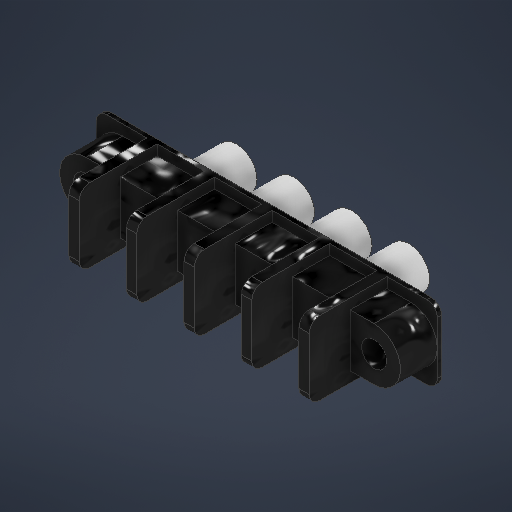
# Autodesk Inventor part: 52160004A
Saved by Autodesk Inventor 2026.2 (Build 302298010, 298A)
## iProperties
Created: 2026-08-03
Part Number: 52160004A
Material: Generic
Document SubType Name: Modeling
Designer: sonata
Density: 1 g/cm^3
Appearance: Default
Author: sonata
Autodesk Inventor part; units mm, degrees
ref_plane "YZ Plane" through (0, 0, 0) normal (1, 0, 0) x (0, 1, 0)
ref_plane "XZ Plane" through (0, 0, 0) normal (0, 1, 0) x (-1, 0, 0)
ref_plane "XY Plane" through (0, 0, 0) normal (0, 0, 1) x (1, 0, 0)
sketch "Sketch1" plane through (0, 0, 0) normal (0, 0, 1) x (1, 0, 0)
  line L0 (0, 0) -> (65.8, 0)
  line L1 (65.8, 0) -> (65.8, 14.2)
  line L2 (65.8, 14.2) -> (0, 14.2)
  line L3 (0, 14.2) -> (0, 0)
  dimension "d0" = 65.8
  dimension "d1" = 14.2
  constraints: 8 end point, 2 parallel, 1 coincident, 1 horizontal, 1 perpendicular
  measures "d0" distance of L1.end L2.end
  measures "d1" distance of L2.end L0.start
extrude "Extrusion1" add sketch "Sketch1" along normal blind 0.81
fillet "Fillet1" radius 2 4 edges at (0, 14.2, 0.405) (65.8, 14.2, 0.405) (65.8, 0, 0.405) (0, 0, 0.405)
sketch "Sketch2" plane through (0, 0, 0.81) normal (0, 0, 1) x (1, 0, 0)
  circle A0 centre (5.1, 7.1) radius 5.1
  line L0 (0, 12.2) -> (0, 2) projected
  circle A1 centre (60.7, 7.1) radius 5.1
  line L1 (65.8, 2) -> (65.8, 12.2) projected
  line L2 (5.1, 12.2) -> (60.7, 12.2)
  line L3 (60.7, 2) -> (5.1, 2)
  point P0 (0, 0)
  point P1 (0, 7.1)
  dimension "d5" = 10.2
  dimension "d6" = 10.2
  constraints: 5 tangent, 4 end point, 4 point on circle, 2 centre point, 2 horizontal alignment, 1 midpoint, 1 parallel
  measures "d5" diameter of A0
  measures "d6" diameter of A1
extrude "Extrusion2" add sketch "Sketch2" along normal blind 7.11
sketch "Sketch3" plane through (0, 0, 7.92) normal (0, 0, 1) x (1, 0, 0)
  line L0 (2, 0) -> (63.8, 0) projected
  line L1 (32.9, 0) -> (32.9, 14.2) construction
  line L2 (63.8, 14.2) -> (2, 14.2) projected
  circle A0 centre (5.1, 7.1) radius 2.4
  circle A1 centre (60.7, 7.1) radius 2.4
  line L3 (5.1, 7.1) -> (60.7, 7.1) construction
  point P0 (0, 0)
  dimension "d9" = 4.8
  dimension "d10" = 4.8
  dimension "d12" = 27.8
  dimension "d13" = 27.8
  dimension "d14" = 7.1
  constraints: 4 end point, 2 centre point, 2 midpoint, 1 horizontal
  measures "d9" diameter of A0
  measures "d10" diameter of A1
  measures "d12" distance from line of L1 L3.start
  measures "d13" distance from line of L3.end L1
  measures "d14" distance between parallel lines of L0 L3
extrude "Extrusion3" cut sketch "Sketch3" against normal through all
sketch "Sketch4" plane through (0, 0, 7.92) normal (0, 0, 1) x (1, 0, 0)
  line L0 (63.8, 14.2) -> (2, 14.2) projected
  line L1 (32.9, 14.2) -> (32.9, 0) construction
  line L2 (2, 0) -> (63.8, 0) projected
  line L3 (31.9, 14.2) -> (33.9, 14.2)
  line L4 (33.9, 14.2) -> (33.9, 0)
  line L5 (33.9, 0) -> (31.9, 0)
  line L6 (31.9, 0) -> (31.9, 14.2)
  line L7 (20.8, 14.2) -> (22.8, 14.2)
  line L8 (22.8, 14.2) -> (22.8, 0)
  line L9 (22.8, 0) -> (20.8, 0)
  line L10 (20.8, 0) -> (20.8, 14.2)
  line L11 (11.7, 0) -> (9.7, 0)
  line L12 (9.7, 0) -> (9.7, 14.2)
  line L13 (9.7, 14.2) -> (11.7, 14.2)
  line L14 (11.7, 14.2) -> (11.7, 0)
  line L15 (43, 14.2) -> (45, 14.2)
  line L16 (45, 14.2) -> (45, 0)
  line L17 (45, 0) -> (43, 0)
  line L18 (43, 0) -> (43, 14.2)
  line L19 (54.1, 0) -> (56.1, 0)
  line L20 (56.1, 0) -> (56.1, 14.2)
  line L21 (56.1, 14.2) -> (54.1, 14.2)
  line L22 (54.1, 14.2) -> (54.1, 0)
  point P0 (0, 0)
  dimension "d17" = 2
  dimension "d18" = 1
  dimension "d19" = 2
  dimension "d20" = 11.1
  dimension "d21" = 11.1
  dimension "d22" = 2
  dimension "d23" = 2
  dimension "d24" = 11.1
  dimension "d25" = 2
  dimension "d26" = 11.1
  constraints: 42 end point, 10 parallel, 10 point on line, 5 horizontal, 5 perpendicular, 2 midpoint
  measures "d17" distance between parallel lines of L4 L6
  measures "d18" distance between parallel lines of L4 L1
  measures "d19" distance between parallel lines of L10 L8
  measures "d20" distance between parallel lines of L4 L8
  measures "d21" distance between parallel lines of L8 L14
  measures "d22" distance between parallel lines of L14 L12
  measures "d23" distance between parallel lines of L16 L18
  measures "d24" distance between parallel lines of L18 L6
  measures "d25" distance between parallel lines of L20 L22
  measures "d26" distance between parallel lines of L22 L18
extrude "Extrusion4" add sketch "Sketch4" along normal mid plane 15.8 contours L20 L2 L22 L0 | L16 L2 L18 L0 | L4 L2 L6 L0 | L8 L2 L10 L0 | L14 L2 L12 L0
fillet "Fillet2" radius 2 10 edges at (10.7, 14.2, 15.82) (21.8, 14.2, 15.82) (32.9, 14.2, 15.82) (44, 14.2, 15.82) (55.1, 14.2, 15.82) (55.1, 0, 15.82) (44, 0, 15.82) (32.9, 0, 15.82) (21.8, 0, 15.82) (10.7, 0, 15.82)
sketch "Sketch5" plane through (0, 0, 0) normal (0, 0, -1) x (-1, 0, 0)
  arc A0 (-65.8, 7.1) -> (-60.7, 2) centre (-60.7, 7.1) ccw projected
  line L0 (0, 7.1) -> (0, 2) projected
  line L1 (-65.8, 7.1) -> (0, 7.1) construction
  circle A1 centre (-38.45, 7.1) radius 3.95
  circle A2 centre (-49.55, 7.1) radius 3.95
  circle A3 centre (-27.35, 7.1) radius 3.95
  circle A4 centre (-16.25, 7.1) radius 3.95
  line L2 (-2, 0) -> (-63.8, 0) projected
  line L3 (-32.9, 0) -> (-32.9, 14.1224) construction
  line L4 (-31.9, 2) -> (-31.9, 12.2) projected
  point P0 (0, 0)
  dimension "d30" = 7.9
  dimension "d31" = 7.9
  dimension "d32" = 7.9
  dimension "d33" = 7.9
  dimension "d34" = 5.55
  dimension "d35" = 5.55
  dimension "d36" = 11.1
  dimension "d37" = 11.1
  constraints: 4 centre point, 4 end point, 4 point on line, 1 horizontal, 1 midpoint, 1 parallel
  measures "d30" diameter of A1
  measures "d31" diameter of A3
  measures "d32" diameter of A4
  measures "d33" diameter of A2
  measures "d34" distance from line of L3 A1.centre
  measures "d35" distance from line of A3.centre L3
  measures "d36" distance of A4.centre A3.centre
  measures "d37" distance of A1.centre A2.centre
extrude "Extrusion5" add sketch "Sketch5" along normal blind 10
body "Solid1"
